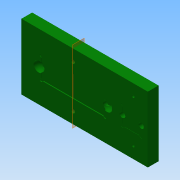
# Autodesk Inventor part: DPX Slide Jig
Saved by Autodesk Inventor 2015 SP1 (Build 190203100, 203)
## iProperties
Created: 2014-11-06
Material: DELRIN 100, BLACK (EXTRUDED)
Vendor: HHMI: JFRC - ID&F
Document SubType Name: Modeling
Designer: KLOSSR
Density: 1.42 g/cm^3
Mass: 205.473 g
Surface Area: 299.959 cm^2
Volume: 144.699 cm^3
Appearance: Dark Green
RuleStatus: InUse
AfterDocSave0: file://Part Number Cleaner
DESIGN DEPARTMENT: HHMI: JFRC - ID&F
ALTERED ITEM PART NUMBER: N/A
ALTERED ITEM VENDOR: N/A
ALTERED ITEM DESCRIPTION: N/A
Author: KLOSSR
Revision Number: 0
Autodesk Inventor part; units mm, degrees
ref_plane "YZ Plane" through (0, 0, 0) normal (1, 0, 0) x (0, 1, 0)
sketch "Sketch1" plane through (0, 0, 0) normal (0, 0, 1) x (1, 0, 0)
  line L0 (-74.93, 38.9255) -> (74.93, 38.9255)
  line L1 (74.93, 38.9255) -> (74.93, -38.9255)
  line L2 (74.93, -38.9255) -> (-74.93, -38.9255)
  line L3 (-74.93, -38.9255) -> (-74.93, 38.9255)
  point P0 (0, 0)
  point P1 (0, 38.9255)
  point P2 (-74.93, 0)
  dimension "d0" = 149.86
  dimension "d1" = 77.851
  constraints: 8 end point, 2 midpoint, 2 parallel, 1 horizontal, 1 horizontal alignment, 1 perpendicular, 1 vertical alignment
  measures "d0" distance of L0.start L0.end
  measures "d1" distance of L0.end L1.end
extrude "Extrusion1" add sketch "Sketch1" against normal blind 12.7
sketch "Sketch3" plane through (0, 0, 0) normal (0, 0, 1) x (1, 0, 0)
  line L0 (-74.93, -38.9255) -> (-74.93, 38.9255) projected
  line L1 (-51.816, 12.6746) -> (23.9268, 12.6746)
  line L2 (23.9268, 12.6746) -> (23.9268, -12.6746)
  line L3 (23.9268, -12.6746) -> (-51.816, -12.6746)
  line L4 (-51.816, -12.6746) -> (-51.816, 12.6746)
  line L5 (-74.93, -38.9255) -> (-74.93, 38.9255) projected
  line L6 (-74.93, 38.9255) -> (74.93, 38.9255) projected
  line L7 (74.93, 38.9255) -> (74.93, -38.9255) projected
  line L8 (74.93, -38.9255) -> (-74.93, -38.9255) projected
  line L9 (-104.902, 0) -> (104.902, 0) projected
  point P0 (0, 0)
  point P1 (23.9268, 0)
  dimension "d4" = 75.7428
  dimension "d5" = 25.3492
  dimension "d6" = 23.114
  constraints: 8 end point, 2 parallel, 1 horizontal, 1 midpoint, 1 perpendicular, 1 point on line
  measures "d4" distance of L1.start L1.end
  measures "d5" distance of L3.end L1.start
  measures "d6" distance between parallel lines of L4 L0
sketch "Sketch4" plane through (0, 0, 0) normal (0, 0, 1) x (1, 0, 0)
  line L0 (44.7294, 11.176) -> (67.0814, 11.176)
  line L1 (67.0814, 11.176) -> (67.0814, -11.176)
  line L2 (67.0814, -11.176) -> (44.7294, -11.176)
  line L3 (44.7294, -11.176) -> (44.7294, 11.176)
  line L4 (23.9268, 12.6746) -> (23.9268, -12.6746) projected
  line L5 (-104.902, 0) -> (104.902, 0) projected
  point P0 (0, 0)
  point P1 (67.0814, 0)
  dimension "d7" = 22.352
  dimension "d8" = 22.352
  dimension "d9" = 20.8026
  constraints: 8 end point, 2 parallel, 1 horizontal, 1 midpoint, 1 perpendicular, 1 point on line
  measures "d7" distance between parallel lines of L3 L1
  measures "d8" distance between parallel lines of L2 L0
  measures "d9" distance between parallel lines of L4 L3
extrude "Extrusion2" cut sketch "Sketch3" against normal blind 1.016 contours L9 L2 L3 L4 | L4 L1 L2 L9
extrude "Extrusion3" cut sketch "Sketch4" against normal blind 0.254
sketch "Sketch7" plane through (0, 0, 0) normal (0, 0, 1) x (1, 0, 0)
  line L0 (44.7294, -11.176) -> (44.7294, 11.176) projected
  line L1 (67.0814, -11.176) -> (44.7294, -11.176) projected
  line L2 (44.7294, 11.176) -> (44.7294, -11.176) projected
  line L3 (44.7294, -11.176) -> (67.0814, -11.176) projected
  line L4 (67.0814, -11.176) -> (67.0814, 11.176) projected
  line L5 (67.0814, 11.176) -> (44.7294, 11.176) projected
  line L6 (43.5171, -9.9637) -> (45.3131, -8.1676)
  line L7 (45.9417, -12.3883) -> (47.7378, -10.5923)
  line L8 (45.3131, -8.1676) -> (47.7378, -10.5923)
  arc A0 (43.5171, -9.9637) -> (45.9417, -12.3883) centre (44.7294, -11.176) ccw
  point P0 (0, 0)
  dimension "d19" = 45
  dimension "d20" = 2.54
  dimension "d22" = 3.429
  constraints: 6 end point, 2 point on circle, 2 tangent, 1 centre point, 1 coincident, 1 parallel, 1 perpendicular
  measures "d19" angle of L7 L1
  measures "d20" distance from line of L0.start L8
  measures "d22" diameter of A0
extrude "Extrusion5" cut sketch "Sketch7" against normal blind 0.254 contours L1 L7 A0 L6 L0 | L0 L6 L8 L7 L1
sketch "Sketch6" plane through (0, 0, 0) normal (0, 0, 1) x (1, 0, 0)
  line L0 (-51.816, -12.6746) -> (-51.816, 12.6746) projected
  line L1 (23.9268, -12.6746) -> (-51.816, -12.6746) projected
  arc A0 (-53.0283, -11.4623) -> (-50.6037, -13.8869) centre (-51.816, -12.6746) ccw
  line L2 (-53.0283, -11.4623) -> (-51.2323, -9.6662)
  line L3 (-50.6037, -13.8869) -> (-48.8076, -12.0909)
  line L4 (-51.2323, -9.6662) -> (-48.8076, -12.0909)
  point P0 (0, 0)
  dimension "d14" = 3.429
  dimension "d17" = 45
  dimension "d18" = 2.54
  constraints: 6 end point, 2 point on circle, 2 tangent, 1 centre point, 1 coincident, 1 parallel, 1 perpendicular
  measures "d14" diameter of A0
  measures "d17" angle of L3 L1
  measures "d18" distance from line of L4 L0.start
extrude "Extrusion4" cut sketch "Sketch6" against normal blind 1.016
ref_plane "Work Plane1" through (-13.9446, -12.6746, 0) normal (-1, 0, 0) x (0, 0, 1)
ref_plane "Work Plane2" through (55.9054, -11.176, 0) normal (-1, 0, 0) x (0, 0, 1)
mirror "Mirror1" about plane through (-13.9446, -12.6746, 0) normal (-1, 0, 0) of "Extrusion4"
mirror "Mirror2" about plane through (0, 0, 0) normal (0, 1, 0) of "Extrusion4", "Mirror1"
mirror "Mirror3" about plane through (55.9054, -11.176, 0) normal (-1, 0, 0) of "Extrusion5"
mirror "Mirror4" about plane through (0, 0, 0) normal (0, 1, 0) of "Extrusion5", "Mirror3"
sketch "Sketch11" plane through (0, 0, 0) normal (0, 0, 1) x (1, 0, 0)
  line L0 (-51.816, -10.2499) -> (-51.816, 10.2499) projected
  line L1 (-104.902, 0) -> (104.902, 0) projected
  point P0 (23.9268, 3.1623)
  point P1 (-51.816, 3.1623)
  point P2 (0, 0)
  point P3 (-54.483, 0)
  dimension "d44" = 2.667
  constraints: 1 point on line
  measures "d44" distance from line of L0 point (-54.483, 0)
hole "Hole3" at (-54.483, 0, 0) direction (0, 0, -1) diameter 12.192 depth 5.08
fillet "Fillet2" radius 6.096 1 edges at (-54.483, 6.096, -5.08)
mirror "Mirror5" about plane through (-13.9446, -12.6746, 0) normal (-1, 0, 0) of "Hole3", "Fillet2"
sketch "Sketch12" plane through (0, 0, 0) normal (0, 0, 1) x (1, 0, 0)
  line L0 (-51.816, 5.4816) -> (-51.816, 10.2499) projected
  line L1 (23.9268, 10.2499) -> (23.9268, -10.2499) projected
  line L2 (67.0814, 8.7513) -> (67.0814, -8.7513) projected
  line L3 (44.7294, -8.7513) -> (44.7294, 8.7513) projected
  line L4 (-104.902, 0) -> (104.902, 0) projected
  point P0 (23.9268, 5.3506)
  point P1 (0, 0)
  point P2 (-51.816, 0)
  point P3 (23.9268, 0)
  point P4 (44.7294, 0)
  point P5 (67.0814, 0)
  point P6 (67.0814, 0)
  point P7 (44.7294, 0)
  dimension "d53" = 0
  dimension "d54" = 0
  constraints: 2 coincident, 2 midpoint, 2 point on line
  measures "d53" distance from line of point (23.927, 0) L1
  measures "d54" distance from line of L0 point (-51.816, 0)
hole "Hole4" at (-51.816, 0, 0) at (23.9268, 0, 0) at (44.7294, 0, 0) at (67.0814, 0, 0) direction (0, 0, -1) diameter 6.3246 depth 5.08
sketch "Sketch13" plane through (0, 0, 0) normal (0, 0, 1) x (1, 0, 0)
  line L0 (-13.9446, -57.8337) -> (-13.9446, 74.524) projected
  line L1 (-104.902, 0) -> (104.902, 0) projected
  point P0 (0, 0)
  point P1 (-13.9446, 25.4)
  point P2 (-13.9446, -25.4)
  dimension "d63" = 25.4
  dimension "d64" = 25.4
  constraints: 2 point on line
  measures "d63" distance from line of L1 point (-13.945, 25.4)
  measures "d64" distance from line of L1 point (-13.945, -25.4)
sketch "Sketch14" plane through (0, 0, 0) normal (0, 0, 1) x (1, 0, 0)
  line L0 (-104.902, 0) -> (104.902, 0) projected
  line L1 (57.4929, 25.4) -> (57.4929, -25.4)
  line L2 (64.6567, 11.176) -> (47.1541, 11.176) projected
  point P0 (0, 0)
  point P1 (55.9054, 11.176)
  dimension "d65" = 25.4
  dimension "d66" = 25.4
  dimension "d81" = 1.5875
  constraints: 2 end point, 1 midpoint, 1 vertical
  measures "d65" distance from line of L0 L1.start
  measures "d66" distance from line of L0 L1.end
  measures "d81" distance from line of L1 point (55.905, 11.176)
hole "Hole5" at (-13.9446, 25.4, 0) at (-13.9446, -25.4, 0) direction (0, 0, -1) diameter 4.7625 depth 5.08 tip angle 118
hole "Hole6" at (57.4929, 25.4, 0) at (57.4929, -25.4, 0) direction (0, 0, -1) diameter 3.175 depth 5.08 tip angle 118
ref_plane "Work Plane3" through (-13.9446, -12.6746, 0) normal (-1, 0, 0) x (0, 0, 1)
body "Solid1"
